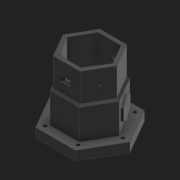
# Autodesk Inventor part: TARM15
Saved by Autodesk Inventor 2017 (Build 210142000, 142)
## iProperties
Created: 2019-07-18
Part Number: TARM15
Material: ABS Plastic
Document SubType Name: Modeling
Designer: Dell
Density: 1.06 g/cm^3
Appearance: Smooth - Black
Author: Dell
Autodesk Inventor part; units mm, degrees
ref_plane "YZ Plane" through (0, 0, 0) normal (1, 0, 0) x (0, 1, 0)
sketch "Sketch1" plane through (0, 0, 0) normal (0, 0, 1) x (1, 0, 0)
  circle A0 centre (0, 0) radius 12.5
  circle A1 centre (51, 0) radius 3
  circle A2 centre (25.5, 44.1673) radius 3
  circle A3 centre (-25.5, 44.1673) radius 3
  circle A4 centre (-51, 0) radius 3
  circle A5 centre (-25.5, -44.1673) radius 3
  circle A6 centre (25.5, -44.1673) radius 3
  line L0 (57.5, 0) -> (28.75, -49.7965)
  line L1 (28.75, -49.7965) -> (-28.75, -49.7965)
  line L2 (-28.75, -49.7965) -> (-57.5, 0)
  line L3 (-57.5, 0) -> (-28.75, 49.7965)
  line L4 (-28.75, 49.7965) -> (28.75, 49.7965)
  line L5 (28.75, 49.7965) -> (57.5, 0)
  line L6 (-30.4821, 52.7965) -> (-60.9641, 0)
  line L7 (-60.9641, 0) -> (-30.4821, -52.7965)
  line L8 (-30.4821, -52.7965) -> (30.4821, -52.7965)
  line L9 (30.4821, -52.7965) -> (60.9641, 0)
  line L10 (60.9641, 0) -> (30.4821, 52.7965)
  line L11 (30.4821, 52.7965) -> (-30.4821, 52.7965)
  dimension "d0" = 25
  dimension "d1" = 6
  dimension "d2" = 51
  dimension "d5" = 360
  dimension "d7" = 115
  dimension "d8" = 3
  constraints: 24 end point, 7 centre point, 2 coincident, 2 horizontal alignment, 31 other
  measures "d0" diameter of A0
  measures "d1" diameter of A1
  measures "d2" distance of A1.centre point (0, 0)
  measures "d7" distance of L0.start L2.end
  measures "d8" distance between parallel lines of L3 L6
extrude "Extrusion1" add sketch "Sketch1" along normal blind 10 contours L0 L1 L2 L3 L4 L5 | L11 L10 L9 L8 L7 L6
sketch "Sketch2" plane through (0, 0, 0) normal (0, 0, -1) x (-1, 0, 0)
  circle A0 centre (0, 0) radius 12.5 projected
  circle A1 centre (-25.5, -44.1673) radius 3 projected
  circle A2 centre (25.5, -44.1673) radius 3 projected
  circle A3 centre (51, 0) radius 3 projected
  circle A4 centre (25.5, 44.1673) radius 3 projected
  circle A5 centre (-25.5, 44.1673) radius 3 projected
  circle A6 centre (-51, 0) radius 3 projected
  line L0 (30.4821, 52.7965) -> (60.9641, 0) projected
  line L1 (-30.4821, 52.7965) -> (30.4821, 52.7965) projected
  line L2 (-60.9641, 0) -> (-30.4821, 52.7965) projected
  line L3 (-30.4821, -52.7965) -> (-60.9641, 0) projected
  line L4 (30.4821, -52.7965) -> (-30.4821, -52.7965) projected
  line L5 (60.9641, 0) -> (30.4821, -52.7965) projected
  line L6 (36.2556, -62.7965) -> (-36.2556, -62.7965)
  line L7 (-36.2556, -62.7965) -> (-72.5111, 0)
  line L8 (-72.5111, 0) -> (-36.2556, 62.7965)
  line L9 (-36.2556, 62.7965) -> (36.2556, 62.7965)
  line L10 (36.2556, 62.7965) -> (72.5111, 0)
  line L11 (72.5111, 0) -> (36.2556, -62.7965)
  dimension "d11" = 10
  constraints: 12 end point, 5 other
  measures "d11" distance between parallel lines of L5 L11
extrude "Extrusion2" add sketch "Sketch2" against normal blind 85 contours L6 L7 L8 L9 L10 L11
ref_plane "Work Plane1" through (0, 0, 35) normal (0, 0, -1) x (-1, 0, 0)
sketch "Sketch4" plane through (0, 0, 35) normal (0, 0, -1) x (-1, 0, 0)
  line L0 (36.2556, -62.7965) -> (-36.2556, -62.7965) projected
  line L1 (19.7879, -62.7965) -> (14.0144, -52.7965)
  line L2 (30.4821, -52.7965) -> (-30.4821, -52.7965) projected
  line L3 (-14.8536, -52.7965) -> (14.0144, -52.7965)
  line L4 (-14.8536, -52.7965) -> (-9.0801, -62.7965)
  line L5 (-9.0801, -62.7965) -> (19.7879, -62.7965)
  point P0 (0, 0)
  point P1 (11.6009, -5.3708)
  dimension "d28" = 60
  dimension "d29" = 28.868
  dimension "d30" = 21.402
  constraints: 8 end point, 4 point on line, 2 collinear, 1 parallel, 4 other
  measures "d28" angle of L5 L1
  measures "d29" distance of L1.end L3.start
  measures "d30" horizontal distance of L2.end L4.end
extrude "Extrusion4" cut sketch "Sketch4" against normal blind 15
ref_plane "Work Plane2" through (-36.2556, -62.7965, 85) normal (-0.5, 0.866, 0) x (0.866, 0.5, 0)
sketch "Sketch5" plane through (-36.2556, -62.7965, 85) normal (-0.5, 0.866, 0) x (0.866, 0.5, 0)
  line L0 (125.5929, 85) -> (125.5929, 0) projected
  circle A0 centre (97.5929, 40) radius 3
  line L1 (115.5929, 75) -> (62.7965, 75) projected
  point P0 (0, 0)
  dimension "d38" = 6
  dimension "d39" = 35
  dimension "d40" = 28
  constraints: 1 centre point
  measures "d38" diameter of A0
  measures "d39" distance from line of L1 A0.centre
  measures "d40" distance from line of L0 A0.centre
extrude "Extrusion5" cut sketch "Sketch5" along normal through all both and the other way through all
sketch "Sketch7" plane through (0, 0, 0) normal (0, 0, -1) x (-1, 0, 0)
  line L0 (36.2556, -62.7965) -> (-36.2556, -62.7965) projected
  line L1 (72.5111, 0) -> (36.2556, -62.7965) projected
  line L2 (36.2556, 62.7965) -> (72.5111, 0) projected
  line L3 (-36.2556, 62.7965) -> (36.2556, 62.7965) projected
  line L4 (-72.5111, 0) -> (-36.2556, 62.7965) projected
  line L5 (-36.2556, -62.7965) -> (-72.5111, 0) construction
  circle A0 centre (0, 0) radius 12.5 projected
  circle A1 centre (-25.5, -44.1673) radius 3 projected
  circle A2 centre (25.5, -44.1673) radius 3 projected
  circle A3 centre (51, 0) radius 3 projected
  circle A4 centre (25.5, 44.1673) radius 3 projected
  circle A5 centre (-25.5, 44.1673) radius 3 projected
  circle A6 centre (-51, 0) radius 3 projected
  line L6 (-60.9641, 0) -> (-30.4821, 52.7965) projected
  line L7 (-30.4821, -52.7965) -> (-60.9641, 0) construction
  line L8 (30.4821, -52.7965) -> (-30.4821, -52.7965) projected
  line L9 (60.9641, 0) -> (30.4821, -52.7965) projected
  line L10 (30.4821, 52.7965) -> (60.9641, 0) projected
  line L11 (-30.4821, 52.7965) -> (30.4821, 52.7965) projected
  line L12 (-78.2846, 0) -> (-39.1423, 67.7965)
  line L13 (-39.1423, 67.7965) -> (39.1423, 67.7965)
  line L14 (39.1423, 67.7965) -> (78.2846, 0)
  line L15 (78.2846, 0) -> (39.1423, -67.7965)
  line L16 (39.1423, -67.7965) -> (-39.1423, -67.7965)
  line L17 (-39.1423, -67.7965) -> (-78.2846, 0)
  line L18 (-33.3688, 57.7965) -> (-66.7376, 0)
  line L19 (-66.7376, 0) -> (-33.3688, -57.7965)
  line L20 (-33.3688, -57.7965) -> (33.3688, -57.7965)
  line L21 (33.3688, -57.7965) -> (66.7376, 0)
  line L22 (66.7376, 0) -> (33.3688, 57.7965)
  line L23 (33.3688, 57.7965) -> (-33.3688, 57.7965)
  dimension "d41" = 5
  dimension "d42" = 5
  constraints: 24 end point, 1 coincident, 1 horizontal alignment, 18 other
  measures "d41" distance between parallel lines of L12 L4
  measures "d42" distance between parallel lines of L6 L18
extrude "Extrusion6" add sketch "Sketch7" along normal blind 100 and the other way blind 10 contours L12 L13 L14 L15 L16 L17
sketch "Sketch8" plane through (0, 0, -100) normal (0, 0, -1) x (-1, 0, 0)
  circle A0 centre (-88.2846, 0) radius 4.5
  circle A1 centre (-44.1423, -76.4567) radius 4.5
  circle A2 centre (44.1423, -76.4567) radius 4.5
  circle A3 centre (88.2846, 0) radius 4.5
  circle A4 centre (44.1423, 76.4567) radius 4.5
  circle A5 centre (-44.1423, 76.4567) radius 4.5
  line L0 (-33.3688, 57.7965) -> (33.3688, 57.7965) construction
  line L1 (33.3688, 57.7965) -> (66.7376, 0) construction
  line L2 (66.7376, 0) -> (33.3688, -57.7965) construction
  line L3 (33.3688, -57.7965) -> (-33.3688, -57.7965) construction
  line L4 (-33.3688, -57.7965) -> (-66.7376, 0) construction
  line L5 (-66.7376, 0) -> (-33.3688, 57.7965) construction
  line L6 (-39.1423, 67.7965) -> (-78.2846, 0) projected
  line L7 (-78.2846, 0) -> (-39.1423, -67.7965) projected
  line L8 (-39.1423, -67.7965) -> (39.1423, -67.7965) projected
  line L9 (39.1423, -67.7965) -> (78.2846, 0) projected
  line L10 (78.2846, 0) -> (39.1423, 67.7965) projected
  line L11 (39.1423, 67.7965) -> (-39.1423, 67.7965) projected
  line L12 (-53.5761, -92.7965) -> (-107.1521, 0)
  line L13 (-107.1521, 0) -> (-53.5761, 92.7965)
  line L14 (-53.5761, 92.7965) -> (53.5761, 92.7965)
  line L15 (53.5761, 92.7965) -> (107.1521, 0)
  line L16 (107.1521, 0) -> (53.5761, -92.7965)
  line L17 (53.5761, -92.7965) -> (-53.5761, -92.7965)
  point P0 (0, 0)
  dimension "d47" = 9
  dimension "d48" = 10
  dimension "d51" = 360
  dimension "d53" = 25
  constraints: 12 end point, 6 centre point, 1 horizontal alignment, 18 other
  measures "d47" diameter of A0
  measures "d48" distance of A0.centre point (-78.285, 0)
  measures "d53" distance between parallel lines of L7 L12
extrude "Extrusion7" add sketch "Sketch8" against normal blind 25
sketch "Sketch9" plane through (0, 0, -100) normal (0, 0, -1) x (-1, 0, 0)
  line L0 (33.3688, -57.7965) -> (-33.3688, -57.7965) projected
  line L1 (-15, -57.7965) -> (15, -57.7965)
  line L2 (15, -57.7965) -> (15, -67.7965)
  line L3 (15, -67.7965) -> (-15, -67.7965)
  line L4 (-15, -67.7965) -> (-15, -57.7965)
  line L5 (33.3688, 57.7965) -> (-33.3688, 57.7965) projected
  line L6 (-15, 57.7965) -> (15, 57.7965)
  line L7 (15, 57.7965) -> (15, 67.7965)
  line L8 (15, 67.7965) -> (-15, 67.7965)
  line L9 (-15, 67.7965) -> (-15, 57.7965)
  line L10 (-33.3688, 57.7965) -> (33.3688, 57.7965) projected
  point P0 (0, 0)
  point P1 (0, 57.7965)
  point P2 (0, -57.7965)
  point P3 (0, 57.7965)
  point P4 (0, 57.7965)
  dimension "d56" = 10
  dimension "d57" = 10
  dimension "d58" = 30
  constraints: 16 end point, 4 midpoint, 4 parallel, 3 vertical alignment, 2 horizontal, 2 perpendicular, 2 point on line, 1 coincident
  measures "d56" distance of L6.end L7.end
  measures "d57" distance of L1.end L2.end
  measures "d58" distance of L7.end L8.end
extrude "Extrusion8" cut sketch "Sketch9" against normal blind 10
chamfer "Chamfer1" distance 5 angle 45 6 edges at (-58.7135, 33.8982, 10) (0, 67.7965, 10) (58.7135, 33.8982, 10) (58.7135, -33.8982, 10) (0, -67.7965, 10) (-58.7135, -33.8982, 10)
sketch "Sketch10" plane through (0, 0, -90) normal (0, 0, -1) x (-1, 0, 0)
  line L0 (15, 57.7965) -> (-15, 57.7965) construction
  line L1 (15, 67.7965) -> (15, 57.7965) construction
  line L2 (-15, 67.7965) -> (15, 67.7965) construction
  line L3 (-15, 57.7965) -> (-15, 67.7965) construction
  line L4 (-15, -57.7965) -> (15, -57.7965) construction
  line L5 (-15, -67.7965) -> (-15, -57.7965) construction
  line L6 (15, -67.7965) -> (-15, -67.7965) construction
  line L7 (15, -57.7965) -> (15, -67.7965) construction
  circle A0 centre (0, 62.7965) radius 2.5
  circle A1 centre (0, -62.7965) radius 2.5
  point P0 (0, 0)
  point P1 (0, 67.7965)
  point P2 (0, -57.7965)
  point P3 (-15, 62.7965)
  point P4 (-15, -62.7965)
  dimension "d64" = 5
  dimension "d65" = 5
  constraints: 4 midpoint, 2 centre point, 2 horizontal alignment, 2 vertical alignment
  measures "d64" diameter of A0
  measures "d65" diameter of A1
extrude "Extrusion9" cut sketch "Sketch10" against normal blind 50
sketch "Sketch11" plane through (-78.2846, 0, -75) normal (-0.866, -0.5, 0) x (0, 0, 1)
  line L0 (80, 0) -> (80, -78.2846) projected
  line L1 (0, 0) -> (80, 0) projected
  line L2 (0, 0) -> (0, -78.2846) projected
  line L3 (0, -78.2846) -> (80, -78.2846) projected
  line L4 (50, -21.6423) -> (15, -21.6423)
  line L5 (15, -21.6423) -> (15, -56.6423)
  line L6 (15, -56.6423) -> (50, -56.6423)
  line L7 (50, -56.6423) -> (50, -21.6423)
  circle A0 centre (32.5, -11.6423) radius 1.5
  circle A1 centre (32.5, -66.6423) radius 1.5
  point P0 (75, -39.1423)
  point P1 (50, -39.1423)
  point P2 (80, -39.1423)
  point P3 (32.5, -21.6423)
  point P4 (32.5, -56.6423)
  dimension "d68" = 35
  dimension "d69" = 35
  dimension "d70" = 15
  dimension "d77" = 3
  dimension "d78" = 3
  dimension "d79" = 10
  dimension "d80" = 10
  constraints: 8 end point, 4 midpoint, 2 centre point, 2 parallel, 2 vertical alignment, 1 horizontal, 1 horizontal alignment, 1 perpendicular
  measures "d68" distance of L6.end L5.end
  measures "d69" distance of L5.end L4.end
  measures "d70" distance between parallel lines of L2 L5
  measures "d77" diameter of A0
  measures "d78" diameter of A1
  measures "d79" distance from line of A0.centre L4
  measures "d80" distance from line of L6 A1.centre
extrude "Extrusion10" cut sketch "Sketch11" against normal blind 25 contours L7 L6 L5 L4 | A0 | A1
sketch "Sketch12" plane through (78.2846, 0, 5) normal (0.866, 0.5, 0) x (0, 0, -1)
  line L0 (10, 39.1423) -> (25, 65.1231)
  line L1 (25, 65.1231) -> (55, 65.1231)
  line L2 (55, 65.1231) -> (70, 39.1423)
  line L3 (70, 39.1423) -> (55, 13.1615)
  line L4 (55, 13.1615) -> (25, 13.1615)
  line L5 (25, 13.1615) -> (10, 39.1423)
  line L6 (0, 0) -> (0, 78.2846) projected
  line L7 (80, -14.4338) -> (80, 92.7184) projected
  point P0 (5, 39.1423)
  point P1 (40, 39.1423)
  point P2 (0, 39.1423)
  dimension "d73" = 60
  dimension "d74" = 40
  constraints: 12 end point, 2 horizontal alignment, 1 midpoint, 13 other
  measures "d73" distance of L2.end L0.start
  measures "d74" distance from line of L7 point (40, 39.142)
extrude "Extrusion11" add sketch "Sketch12" along normal blind 5
equation "\"d57\" = d56"
body "Solid1"
